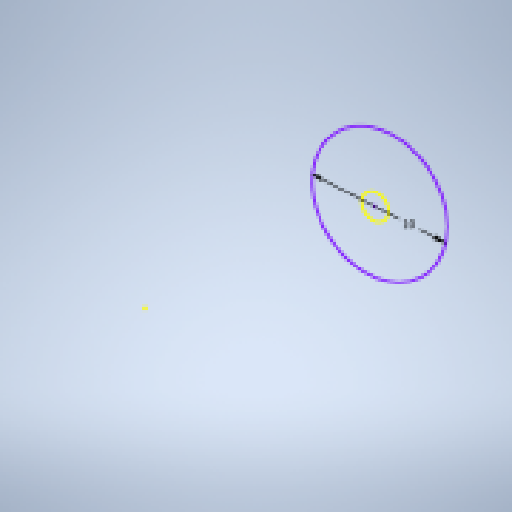
# Autodesk Inventor part: acoplador sensor
Saved by Autodesk Inventor 2023 (Build 270158000, 158)
## iProperties
Created: 2022-10-25
Part Number: acoplador sensor
Material: Generic
Document SubType Name: Modeling
Designer: klebe
Density: 1 g/cm^3
Appearance: Default
Author: klebe
Autodesk Inventor part; units mm, degrees
ref_plane "YZ Plane" through (0, 0, 0) normal (1, 0, 0) x (0, 1, 0)
ref_plane "XZ Plane" through (0, 0, 0) normal (0, 1, 0) x (-1, 0, 0)
ref_plane "XY Plane" through (0, 0, 0) normal (0, 0, 1) x (1, 0, 0)
sketch "Sketch1" plane through (0, 0, 0) normal (0, 0, 1) x (1, 0, 0)
  circle A0 centre (25, 22.275) radius 1 projected
  circle A1 centre (25, 22.275) radius 5
  circle A2 centre (25, 22.275) radius 1
  point P0 (0, 0)
  dimension "d0" = 10
  dimension "d6" = 2
  constraints: 2 centre point, 1 coincident
  measures "d0" diameter of A1
  measures "d6" diameter of A2
extrude "Extrusion1" add sketch "Sketch1" along normal blind 5.5
sketch "Sketch2" plane through (25, 22.275, 5.5) normal (0, 0, 1) x (1, 0, 0)
  circle A0 centre (0, 0) radius 5 projected
  circle A1 centre (0, 0) radius 2.5
  circle A2 centre (0, 0) radius 1
  point P0 (-25, -22.275)
  constraints: 2 centre point, 1 coincident
extrude "Extrusion2" add sketch "Sketch2" along normal blind 16 contours A1
body "Solid1"
